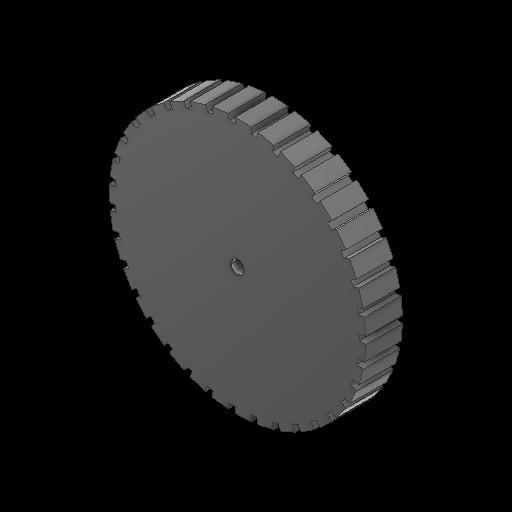
# Autodesk Inventor part: RobotWheelMK1offset
Saved by Autodesk Inventor 2025 (Build 290162000, 162)
## iProperties
Created: 2024-11-18
Part Number: RobotWheelMK1offset
Material: Generic
Document SubType Name: Modeling
Designer: Trevor
Density: 1 g/cm^3
Appearance: Default
Author: Trevor
Autodesk Inventor part; units mm, degrees
ref_plane "YZ Plane" through (0, 0, 0) normal (1, 0, 0) x (0, 1, 0)
ref_plane "XZ Plane" through (0, 0, 0) normal (0, 1, 0) x (-1, 0, 0)
sketch "Sketch1" plane through (0, 0, 0) normal (0, 0, 1) x (1, 0, 0)
  line L0 (-2.4408, -0.5408) -> (-1.2026, 2.1918) projected
  arc A0 (-2.4408, -0.5408) -> (-1.2026, 2.1918) centre (0, 0) ccw projected
  circle A1 centre (0, 0) radius 50
  line L1 (-52.2966, -3.2808) -> (-49.8922, -3.2808)
  line L2 (-49.8922, 3.2808) -> (-52.2966, 3.2808)
  line L3 (-52.2966, 3.2808) -> (-52.2966, -3.2808)
  line L4 (-52.2966, -3.2808) -> (-50, 0) construction
  line L5 (-50, 0) -> (-52.2966, 3.2808) construction
  line L6 (-49.6763, -5.6805) -> (-52.042, -6.1098)
  line L7 (-52.042, -6.1098) -> (-50.8703, -12.566)
  line L8 (-50.8703, -12.566) -> (-48.5046, -12.1367)
  circle A2 centre (0, 0) radius 50
  line L9 (-47.8637, -14.4592) -> (-50.1147, -15.3041)
  line L10 (-50.1147, -15.3041) -> (-47.8091, -21.4473)
  line L11 (-47.8091, -21.4473) -> (-45.5581, -20.6025)
  circle A3 centre (0, 0) radius 50
  line L12 (-44.5127, -22.7733) -> (-46.5767, -24.0064)
  line L13 (-46.5767, -24.0064) -> (-43.2112, -29.6393)
  line L14 (-43.2112, -29.6393) -> (-41.1472, -28.4061)
  circle A4 centre (0, 0) radius 50
  line L15 (-39.731, -30.3553) -> (-41.5417, -31.9372)
  line L16 (-41.5417, -31.9372) -> (-37.2245, -36.8787)
  line L17 (-37.2245, -36.8787) -> (-35.4138, -35.2967)
  circle A5 centre (0, 0) radius 50
  line L18 (-33.6724, -36.9618) -> (-35.1715, -38.8415)
  line L19 (-35.1715, -38.8415) -> (-30.0413, -42.9327)
  line L20 (-30.0413, -42.9327) -> (-28.5422, -41.0529)
  circle A6 centre (0, 0) radius 50
  line L21 (-26.5315, -42.3802) -> (-27.6708, -44.4975)
  line L22 (-27.6708, -44.4975) -> (-21.8926, -47.6068)
  line L23 (-21.8926, -47.6068) -> (-20.7533, -45.4896)
  circle A7 centre (0, 0) radius 50
  line L24 (-18.5378, -46.4365) -> (-19.2808, -48.7232)
  line L25 (-19.2808, -48.7232) -> (-13.0403, -50.7508)
  line L26 (-13.0403, -50.7508) -> (-12.2973, -48.4642)
  circle A8 centre (0, 0) radius 50
  line L27 (-9.9483, -49.0003) -> (-10.2711, -51.3829)
  line L28 (-10.2711, -51.3829) -> (-3.7688, -52.2637)
  line L29 (-3.7688, -52.2637) -> (-3.4461, -49.8811)
  circle A9 centre (0, 0) radius 50
  line L30 (-1.0391, -49.9892) -> (-0.9313, -52.3911)
  line L31 (-0.9313, -52.3911) -> (5.6238, -52.0967)
  line L32 (5.6238, -52.0967) -> (5.5159, -49.6948)
  circle A10 centre (0, 0) radius 50
  line L33 (7.9035, -49.3714) -> (8.4385, -51.7155)
  line L34 (8.4385, -51.7155) -> (14.8357, -50.2553)
  line L35 (14.8357, -50.2553) -> (14.3007, -47.9113)
  circle A11 centre (0, 0) radius 50
  line L36 (16.5921, -47.1668) -> (17.537, -49.3776)
  line L37 (17.537, -49.3776) -> (23.5707, -46.7987)
  line L38 (23.5707, -46.7987) -> (22.6257, -44.5879)
  circle A12 centre (0, 0) radius 50
  line L39 (24.7474, -43.4461) -> (26.0719, -45.4527)
  line L40 (26.0719, -45.4527) -> (31.5481, -41.8379)
  line L41 (31.5481, -41.8379) -> (30.2236, -39.8313)
  circle A13 centre (0, 0) radius 50
  line L42 (32.1073, -38.3291) -> (33.7688, -40.067)
  line L43 (33.7688, -40.067) -> (38.5116, -35.5324)
  line L44 (38.5116, -35.5324) -> (36.85, -33.7946)
  circle A14 centre (0, 0) radius 50
  line L45 (38.4352, -31.9802) -> (40.3804, -33.3934)
  line L46 (40.3804, -33.3934) -> (44.2373, -28.0849)
  line L47 (44.2373, -28.0849) -> (42.2921, -26.6717)
  circle A15 centre (0, 0) radius 50
  line L48 (43.5279, -24.6034) -> (45.6941, -25.6466)
  line L49 (45.6941, -25.6466) -> (48.5411, -19.7347)
  line L50 (48.5411, -19.7347) -> (46.3749, -18.6915)
  circle A16 centre (0, 0) radius 50
  line L51 (47.2214, -16.4358) -> (49.5391, -17.0754)
  line L52 (49.5391, -17.0754) -> (51.2848, -10.7502)
  line L53 (51.2848, -10.7502) -> (48.9671, -10.1106)
  circle A17 centre (0, 0) radius 50
  line L54 (49.3973, -7.7399) -> (51.792, -7.9555)
  line L55 (51.792, -7.9555) -> (52.3801, -1.4202)
  line L56 (52.3801, -1.4202) -> (49.9855, -1.2047)
  circle A18 centre (0, 0) radius 50
  line L57 (49.9855, 1.2047) -> (52.3801, 1.4202)
  line L58 (52.3801, 1.4202) -> (51.792, 7.9555)
  line L59 (51.792, 7.9555) -> (49.3973, 7.7399)
  circle A19 centre (0, 0) radius 50
  line L60 (48.9671, 10.1106) -> (51.2848, 10.7502)
  line L61 (51.2848, 10.7502) -> (49.5391, 17.0754)
  line L62 (49.5391, 17.0754) -> (47.2214, 16.4358)
  circle A20 centre (0, 0) radius 50
  line L63 (46.3749, 18.6915) -> (48.5411, 19.7347)
  line L64 (48.5411, 19.7347) -> (45.6941, 25.6466)
  line L65 (45.6941, 25.6466) -> (43.5279, 24.6034)
  circle A21 centre (0, 0) radius 50
  line L66 (42.2921, 26.6717) -> (44.2373, 28.0849)
  line L67 (44.2373, 28.0849) -> (40.3804, 33.3934)
  line L68 (40.3804, 33.3934) -> (38.4352, 31.9802)
  circle A22 centre (0, 0) radius 50
  line L69 (36.85, 33.7946) -> (38.5116, 35.5324)
  line L70 (38.5116, 35.5324) -> (33.7688, 40.067)
  line L71 (33.7688, 40.067) -> (32.1073, 38.3291)
  circle A23 centre (0, 0) radius 50
  line L72 (30.2236, 39.8313) -> (31.5481, 41.8379)
  line L73 (31.5481, 41.8379) -> (26.0719, 45.4527)
  line L74 (26.0719, 45.4527) -> (24.7474, 43.4461)
  circle A24 centre (0, 0) radius 50
  line L75 (22.6257, 44.5879) -> (23.5707, 46.7987)
  line L76 (23.5707, 46.7987) -> (17.537, 49.3776)
  line L77 (17.537, 49.3776) -> (16.5921, 47.1668)
  circle A25 centre (0, 0) radius 50
  line L78 (14.3007, 47.9113) -> (14.8357, 50.2553)
  line L79 (14.8357, 50.2553) -> (8.4385, 51.7155)
  line L80 (8.4385, 51.7155) -> (7.9035, 49.3714)
  circle A26 centre (0, 0) radius 50
  line L81 (5.5159, 49.6948) -> (5.6238, 52.0967)
  line L82 (5.6238, 52.0967) -> (-0.9313, 52.3911)
  line L83 (-0.9313, 52.3911) -> (-1.0391, 49.9892)
  circle A27 centre (0, 0) radius 50
  line L84 (-3.4461, 49.8811) -> (-3.7688, 52.2637)
  line L85 (-3.7688, 52.2637) -> (-10.2711, 51.3829)
  line L86 (-10.2711, 51.3829) -> (-9.9483, 49.0003)
  circle A28 centre (0, 0) radius 50
  line L87 (-12.2973, 48.4642) -> (-13.0403, 50.7508)
  line L88 (-13.0403, 50.7508) -> (-19.2808, 48.7232)
  line L89 (-19.2808, 48.7232) -> (-18.5378, 46.4365)
  circle A29 centre (0, 0) radius 50
  line L90 (-20.7533, 45.4896) -> (-21.8926, 47.6068)
  line L91 (-21.8926, 47.6068) -> (-27.6708, 44.4975)
  line L92 (-27.6708, 44.4975) -> (-26.5315, 42.3802)
  circle A30 centre (0, 0) radius 50
  line L93 (-28.5422, 41.0529) -> (-30.0413, 42.9327)
  line L94 (-30.0413, 42.9327) -> (-35.1715, 38.8415)
  line L95 (-35.1715, 38.8415) -> (-33.6724, 36.9618)
  circle A31 centre (0, 0) radius 50
  line L96 (-35.4138, 35.2967) -> (-37.2245, 36.8787)
  line L97 (-37.2245, 36.8787) -> (-41.5417, 31.9372)
  line L98 (-41.5417, 31.9372) -> (-39.731, 30.3553)
  circle A32 centre (0, 0) radius 50
  line L99 (-41.1472, 28.4061) -> (-43.2112, 29.6393)
  line L100 (-43.2112, 29.6393) -> (-46.5767, 24.0064)
  line L101 (-46.5767, 24.0064) -> (-44.5127, 22.7733)
  circle A33 centre (0, 0) radius 50
  line L102 (-45.5581, 20.6025) -> (-47.8091, 21.4473)
  line L103 (-47.8091, 21.4473) -> (-50.1147, 15.3041)
  line L104 (-50.1147, 15.3041) -> (-47.8637, 14.4592)
  circle A34 centre (0, 0) radius 50
  line L105 (-48.5046, 12.1367) -> (-50.8703, 12.566)
  line L106 (-50.8703, 12.566) -> (-52.042, 6.1098)
  line L107 (-52.042, 6.1098) -> (-49.6763, 5.6805)
  circle A35 centre (0, 0) radius 50
  line L108 (-1.2026, 2.1918) -> (-2.4408, -0.5408)
  arc A36 (-2.4408, -0.5408) -> (-1.2026, 2.1918) centre (0, 0) ccw
  point P0 (0, 0)
  point P1 (-49.1965, -8.9278)
  point P2 (-46.8117, -17.5687)
  point P3 (-42.9224, -25.645)
  point P4 (-37.6536, -32.8969)
  point P5 (-31.1745, -39.0916)
  point P6 (-23.6934, -44.0298)
  point P7 (-15.4508, -47.5528)
  point P8 (-6.7117, -49.5475)
  point P9 (2.2432, -49.9497)
  point P10 (11.126, -48.7464)
  point P11 (19.6513, -45.9764)
  point P12 (27.5448, -41.7287)
  point P13 (34.5531, -36.1397)
  point P14 (40.4508, -29.3893)
  point P15 (45.0484, -21.6942)
  point P16 (48.1981, -13.3018)
  point P17 (49.7987, -4.482)
  point P18 (49.7987, 4.482)
  point P19 (48.1981, 13.3018)
  point P20 (45.0484, 21.6942)
  point P21 (40.4508, 29.3893)
  point P22 (34.5531, 36.1397)
  point P23 (27.5448, 41.7287)
  point P24 (19.6513, 45.9764)
  point P25 (11.126, 48.7464)
  point P26 (2.2432, 49.9497)
  point P27 (-6.7117, 49.5475)
  point P28 (-15.4508, 47.5528)
  point P29 (-23.6934, 44.0298)
  point P30 (-31.1745, 39.0916)
  point P31 (-37.6536, 32.8969)
  point P32 (-42.9224, 25.645)
  point P33 (-46.8117, 17.5687)
  point P34 (-49.1965, 8.9278)
  dimension "d0" = 100
  dimension "d5" = 360
  dimension "d9" = 0
  constraints: 216 end point, 104 point on circle, 35 centre point, 2 coincident with centre, 1 coincident, 1 horizontal, 1 parallel, 355 other
  measures "d9" radial gap between concentric circles of A0 A36
ref_plane "Work Plane1" through (-2, -2, 15) normal (0, 0, 1) x (1, 0, 0)
extrude "Extrusion1" add sketch "Sketch1" along normal up to surface (15 mm away)
sketch "Sketch2" plane through (-52.2966, -3.2808, 15) normal (0, 0, 1) x (1, 0, 0)
  line L0 (51.094, 5.4726) -> (49.8558, 2.74) projected
  arc A0 (49.8558, 2.74) -> (51.094, 5.4726) centre (52.2966, 3.2808) ccw projected
  line L1 (0.2546, 9.3906) -> (1.4262, 15.8469) projected
  line L2 (2.6203, 8.9613) -> (0.2546, 9.3906) projected
  arc A1 (2.6203, 8.9613) -> (2.4043, 6.5617) centre (52.2966, 3.2808) ccw projected
  line L3 (0, 6.5617) -> (2.4043, 6.5617) projected
  line L4 (0, 0) -> (0, 6.5617) projected
  line L5 (2.4043, 0) -> (0, 0) projected
  arc A2 (2.4043, 0) -> (2.6203, -2.3996) centre (52.2966, 3.2808) ccw projected
  line L6 (0.2546, -2.829) -> (2.6203, -2.3996) projected
  line L7 (1.4262, -9.2852) -> (0.2546, -2.829) projected
  line L8 (3.7919, -8.8559) -> (1.4262, -9.2852) projected
  arc A3 (3.7919, -8.8559) -> (4.4329, -11.1784) centre (52.2966, 3.2808) ccw projected
  line L9 (2.1819, -12.0232) -> (4.4329, -11.1784) projected
  line L10 (4.4875, -18.1665) -> (2.1819, -12.0232) projected
  line L11 (6.7385, -17.3217) -> (4.4875, -18.1665) projected
  arc A4 (6.7385, -17.3217) -> (7.7839, -19.4924) centre (52.2966, 3.2808) ccw projected
  line L12 (5.7199, -20.7256) -> (7.7839, -19.4924) projected
  line L13 (9.0854, -26.3585) -> (5.7199, -20.7256) projected
  line L14 (11.1494, -25.1253) -> (9.0854, -26.3585) projected
  arc A5 (11.1494, -25.1253) -> (12.5656, -27.0745) centre (52.2966, 3.2808) ccw projected
  line L15 (10.7549, -28.6564) -> (12.5656, -27.0745) projected
  line L16 (15.0721, -33.5978) -> (10.7549, -28.6564) projected
  line L17 (16.8828, -32.0159) -> (15.0721, -33.5978) projected
  arc A6 (16.8828, -32.0159) -> (18.6242, -33.6809) centre (52.2966, 3.2808) ccw projected
  line L18 (17.1251, -35.5607) -> (18.6242, -33.6809) projected
  line L19 (22.2553, -39.6518) -> (17.1251, -35.5607) projected
  line L20 (23.7543, -37.7721) -> (22.2553, -39.6518) projected
  arc A7 (23.7543, -37.7721) -> (25.7651, -39.0994) centre (52.2966, 3.2808) ccw projected
  line L21 (24.6258, -41.2166) -> (25.7651, -39.0994) projected
  line L22 (30.404, -44.326) -> (24.6258, -41.2166) projected
  line L23 (31.5433, -42.2087) -> (30.404, -44.326) projected
  arc A8 (31.5433, -42.2087) -> (33.7588, -43.1557) centre (52.2966, 3.2808) ccw projected
  line L24 (33.0158, -45.4423) -> (33.7588, -43.1557) projected
  line L25 (39.2563, -47.47) -> (33.0158, -45.4423) projected
  line L26 (39.9993, -45.1833) -> (39.2563, -47.47) projected
  arc A9 (39.9993, -45.1833) -> (42.3482, -45.7195) centre (52.2966, 3.2808) ccw projected
  line L27 (42.0255, -48.1021) -> (42.3482, -45.7195) projected
  line L28 (48.5278, -48.9828) -> (42.0255, -48.1021) projected
  line L29 (48.8505, -46.6003) -> (48.5278, -48.9828) projected
  arc A10 (48.8505, -46.6003) -> (51.2575, -46.7084) centre (52.2966, 3.2808) ccw projected
  line L30 (51.3653, -49.1103) -> (51.2575, -46.7084) projected
  line L31 (57.9204, -48.8159) -> (51.3653, -49.1103) projected
  line L32 (57.8125, -46.414) -> (57.9204, -48.8159) projected
  arc A11 (57.8125, -46.414) -> (60.2001, -46.0906) centre (52.2966, 3.2808) ccw projected
  line L33 (60.7351, -48.4346) -> (60.2001, -46.0906) projected
  line L34 (67.1323, -46.9745) -> (60.7351, -48.4346) projected
  line L35 (66.5972, -44.6304) -> (67.1323, -46.9745) projected
  arc A12 (66.5972, -44.6304) -> (68.8887, -43.8859) centre (52.2966, 3.2808) ccw projected
  line L36 (69.8336, -46.0968) -> (68.8887, -43.8859) projected
  line L37 (75.8673, -43.5179) -> (69.8336, -46.0968) projected
  line L38 (74.9223, -41.307) -> (75.8673, -43.5179) projected
  arc A13 (74.9223, -41.307) -> (77.044, -40.1653) centre (52.2966, 3.2808) ccw projected
  line L39 (78.3685, -42.1719) -> (77.044, -40.1653) projected
  line L40 (83.8447, -38.5571) -> (78.3685, -42.1719) projected
  line L41 (82.5202, -36.5505) -> (83.8447, -38.5571) projected
  arc A14 (82.5202, -36.5505) -> (84.4039, -35.0483) centre (52.2966, 3.2808) ccw projected
  line L42 (86.0654, -36.7861) -> (84.4039, -35.0483) projected
  line L43 (90.8082, -32.2516) -> (86.0654, -36.7861) projected
  line L44 (89.1466, -30.5138) -> (90.8082, -32.2516) projected
  arc A15 (89.1466, -30.5138) -> (90.7318, -28.6993) centre (52.2966, 3.2808) ccw projected
  line L45 (92.677, -30.1126) -> (90.7318, -28.6993) projected
  line L46 (96.5338, -24.8041) -> (92.677, -30.1126) projected
  line L47 (94.5887, -23.3908) -> (96.5338, -24.8041) projected
  arc A16 (94.5887, -23.3908) -> (95.8244, -21.3225) centre (52.2966, 3.2808) ccw projected
  line L48 (97.9907, -22.3657) -> (95.8244, -21.3225) projected
  line L49 (100.8377, -16.4539) -> (97.9907, -22.3657) projected
  line L50 (98.6715, -15.4107) -> (100.8377, -16.4539) projected
  arc A17 (98.6715, -15.4107) -> (99.518, -13.1549) centre (52.2966, 3.2808) ccw projected
  line L51 (101.8357, -13.7946) -> (99.518, -13.1549) projected
  line L52 (103.5814, -7.4694) -> (101.8357, -13.7946) projected
  line L53 (101.2637, -6.8297) -> (103.5814, -7.4694) projected
  arc A18 (101.2637, -6.8297) -> (101.6939, -4.4591) centre (52.2966, 3.2808) ccw projected
  line L54 (104.0886, -4.6746) -> (101.6939, -4.4591) projected
  line L55 (104.6767, 1.8606) -> (104.0886, -4.6746) projected
  line L56 (102.2821, 2.0762) -> (104.6767, 1.8606) projected
  arc A19 (102.2821, 2.0762) -> (102.2821, 4.4855) centre (52.2966, 3.2808) ccw projected
  line L57 (104.6767, 4.701) -> (102.2821, 4.4855) projected
  line L58 (104.0886, 11.2363) -> (104.6767, 4.701) projected
  line L59 (101.6939, 11.0208) -> (104.0886, 11.2363) projected
  arc A20 (101.6939, 11.0208) -> (101.2637, 13.3914) centre (52.2966, 3.2808) ccw projected
  line L60 (103.5814, 14.0311) -> (101.2637, 13.3914) projected
  line L61 (101.8357, 20.3563) -> (103.5814, 14.0311) projected
  line L62 (99.518, 19.7166) -> (101.8357, 20.3563) projected
  arc A21 (99.518, 19.7166) -> (98.6715, 21.9723) centre (52.2966, 3.2808) ccw projected
  line L63 (100.8377, 23.0155) -> (98.6715, 21.9723) projected
  line L64 (97.9907, 28.9274) -> (100.8377, 23.0155) projected
  line L65 (95.8244, 27.8842) -> (97.9907, 28.9274) projected
  arc A22 (95.8244, 27.8842) -> (94.5887, 29.9525) centre (52.2966, 3.2808) ccw projected
  line L66 (96.5338, 31.3657) -> (94.5887, 29.9525) projected
  line L67 (92.677, 36.6743) -> (96.5338, 31.3657) projected
  line L68 (90.7318, 35.261) -> (92.677, 36.6743) projected
  arc A23 (90.7318, 35.261) -> (89.1466, 37.0754) centre (52.2966, 3.2808) ccw projected
  line L69 (90.8082, 38.8133) -> (89.1466, 37.0754) projected
  line L70 (86.0654, 43.3478) -> (90.8082, 38.8133) projected
  line L71 (84.4039, 41.61) -> (86.0654, 43.3478) projected
  arc A24 (84.4039, 41.61) -> (82.5202, 43.1122) centre (52.2966, 3.2808) ccw projected
  line L72 (83.8447, 45.1188) -> (82.5202, 43.1122) projected
  line L73 (78.3685, 48.7336) -> (83.8447, 45.1188) projected
  line L74 (77.044, 46.727) -> (78.3685, 48.7336) projected
  arc A25 (77.044, 46.727) -> (74.9223, 47.8687) centre (52.2966, 3.2808) ccw projected
  line L75 (75.8673, 50.0796) -> (74.9223, 47.8687) projected
  line L76 (69.8336, 52.6585) -> (75.8673, 50.0796) projected
  line L77 (68.8887, 50.4476) -> (69.8336, 52.6585) projected
  arc A26 (68.8887, 50.4476) -> (66.5972, 51.1921) centre (52.2966, 3.2808) ccw projected
  line L78 (67.1323, 53.5362) -> (66.5972, 51.1921) projected
  line L79 (60.7351, 54.9963) -> (67.1323, 53.5362) projected
  line L80 (60.2001, 52.6522) -> (60.7351, 54.9963) projected
  arc A27 (60.2001, 52.6522) -> (57.8125, 52.9757) centre (52.2966, 3.2808) ccw projected
  line L81 (57.9204, 55.3776) -> (57.8125, 52.9757) projected
  line L82 (51.3653, 55.672) -> (57.9204, 55.3776) projected
  line L83 (51.2575, 53.27) -> (51.3653, 55.672) projected
  arc A28 (51.2575, 53.27) -> (48.8505, 53.1619) centre (52.2966, 3.2808) ccw projected
  line L84 (48.5278, 55.5445) -> (48.8505, 53.1619) projected
  line L85 (42.0255, 54.6637) -> (48.5278, 55.5445) projected
  line L86 (42.3482, 52.2812) -> (42.0255, 54.6637) projected
  arc A29 (42.3482, 52.2812) -> (39.9993, 51.745) centre (52.2966, 3.2808) ccw projected
  line L87 (39.2563, 54.0317) -> (39.9993, 51.745) projected
  line L88 (33.0158, 52.004) -> (39.2563, 54.0317) projected
  line L89 (33.7588, 49.7173) -> (33.0158, 52.004) projected
  arc A30 (33.7588, 49.7173) -> (31.5433, 48.7704) centre (52.2966, 3.2808) ccw projected
  line L90 (30.404, 50.8877) -> (31.5433, 48.7704) projected
  line L91 (24.6258, 47.7783) -> (30.404, 50.8877) projected
  line L92 (25.7651, 45.661) -> (24.6258, 47.7783) projected
  arc A31 (25.7651, 45.661) -> (23.7543, 44.3337) centre (52.2966, 3.2808) ccw projected
  line L93 (22.2553, 46.2135) -> (23.7543, 44.3337) projected
  line L94 (17.1251, 42.1224) -> (22.2553, 46.2135) projected
  line L95 (18.6242, 40.2426) -> (17.1251, 42.1224) projected
  arc A32 (18.6242, 40.2426) -> (16.8828, 38.5776) centre (52.2966, 3.2808) ccw projected
  line L96 (15.0721, 40.1595) -> (16.8828, 38.5776) projected
  line L97 (10.7549, 35.2181) -> (15.0721, 40.1595) projected
  line L98 (12.5656, 33.6362) -> (10.7549, 35.2181) projected
  arc A33 (12.5656, 33.6362) -> (11.1494, 31.687) centre (52.2966, 3.2808) ccw projected
  line L99 (9.0854, 32.9202) -> (11.1494, 31.687) projected
  line L100 (5.7199, 27.2873) -> (9.0854, 32.9202) projected
  line L101 (7.7839, 26.0541) -> (5.7199, 27.2873) projected
  arc A34 (7.7839, 26.0541) -> (6.7385, 23.8834) centre (52.2966, 3.2808) ccw projected
  line L102 (4.4875, 24.7282) -> (6.7385, 23.8834) projected
  line L103 (2.1819, 18.5849) -> (4.4875, 24.7282) projected
  line L104 (4.4329, 17.7401) -> (2.1819, 18.5849) projected
  arc A35 (4.4329, 17.7401) -> (3.7919, 15.4176) centre (52.2966, 3.2808) ccw projected
  line L105 (1.4262, 15.8469) -> (3.7919, 15.4176) projected
  line L106 (49.5946, 2.7693) -> (50.8998, 5.6497)
  arc A36 (49.5946, 2.7693) -> (50.8998, 5.6497) centre (52.2966, 3.2808) ccw
  point P0 (52.2966, 3.2808)
  dimension "d10" = 0.25
  constraints: 2 end point, 2 point on circle, 1 centre point, 1 other
  measures "d10" radial gap between concentric circles of A0 A36
extrude "Extrusion2" cut sketch "Sketch2" against normal up to surface (15 mm away) contours L106 A36
body "Solid1"
